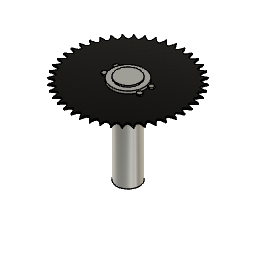
Gear (Autodesk Fusion 360 design; units mm, degrees)
Autodesk Fusion 360 part; units mm, degrees
(part 1 of 4)
sketch "Sketch1" plane through (0, 0, 0) normal (0, 0, 1) x (1, 0, 0)
  line L0 (12.5, 86.6025) -> (12.5, 76.4853)
  line L1 (0, 87.5) -> (0, 77.5)
  spline S0 degree 5 poles (0, 87.5) (0.2426, 86.8577) (0.7286, 85.6271) (1.4594, 83.9437) (2.4376, 82.0293) (3.6674, 80.2243) (4.9048, 79.0612) (6.1503, 78.5945) (7.4045, 78.8575) (8.667, 79.8263) (9.9372, 81.4497) (10.959, 83.23) (11.7283, 84.8192) (12.2426, 85.9896) (12.5, 86.6025) knots 0 0 0 0 0 0 0.1 0.2 0.3 0.4 0.5 0.6 0.7 0.8 0.9 1 1 1 1 1 1
  arc A0 (12.5, 76.4853) -> (0, 77.5) centre (0, 0) ccw
  line L2 (12.5, 89) -> (12.5, 81) construction
  line L3 (6.25, 87.5341) -> (6.25, 78.7707) construction
  arc A1 (1.4878, 77.4857) -> (-11.0294, 76.7112) centre (0, 0) ccw
  line L4 (-12.4525, 86.6094) -> (-11.0294, 76.7112)
  spline S1 degree 5 poles (-12.4525, 86.6094) (-12.121, 86.0081) (-11.4649, 84.8592) (-10.5019, 83.2969) (-9.2612, 81.5413) (-7.787, 79.9297) (-6.3967, 78.9545) (-5.0974, 78.6698) (-3.8935, 79.1086) (-2.7817, 80.2473) (-1.7555, 82.0348) (-0.9974, 83.9425) (-0.4621, 85.6249) (-0.1196, 86.8566) (0.0479, 87.5) knots 0 0 0 0 0 0 0.1 0.2 0.3 0.4 0.5 0.6 0.7 0.8 0.9 1 1 1 1 1 1
  line L5 (0.0479, 87.5) -> (1.4878, 77.4857)
  arc A2 (-9.5547, 76.9088) -> (-21.8343, 74.3607) centre (0, 0) ccw
  line L6 (-24.6516, 83.9556) -> (-21.8343, 74.3607)
  spline S2 degree 5 poles (-24.6516, 83.9556) (-24.2378, 83.4077) (-23.4249, 82.3639) (-22.2494, 80.9545) (-20.7714, 79.3933) (-19.0829, 78.0079) (-17.568, 77.2405) (-16.2414, 77.1436) (-15.1122, 77.7493) (-14.1738, 79.0346) (-13.4124, 80.95) (-12.9335, 82.9461) (-12.6431, 84.6876) (-12.4794, 85.9555) (-12.4051, 86.6162) knots 0 0 0 0 0 0 0.1 0.2 0.3 0.4 0.5 0.6 0.7 0.8 0.9 1 1 1 1 1 1
  line L7 (-12.4051, 86.6162) -> (-9.5547, 76.9088)
  arc A3 (-20.4027, 74.7662) -> (-32.1947, 70.4965) centre (0, 0) ccw
  line L8 (-36.3488, 79.5928) -> (-32.1947, 70.4965)
  spline S3 degree 5 poles (-36.3488, 79.5928) (-35.8613, 79.1093) (-34.9081, 78.1918) (-33.544, 76.9641) (-31.8588, 75.6291) (-29.9904, 74.4981) (-28.3817, 73.9542) (-27.0548, 74.047) (-26.0232, 74.8073) (-25.2773, 76.213) (-24.7963, 78.2173) (-24.6064, 80.2612) (-24.5667, 82.0264) (-24.5851, 83.3046) (-24.6056, 83.9691) knots 0 0 0 0 0 0 0.1 0.2 0.3 0.4 0.5 0.6 0.7 0.8 0.9 1 1 1 1 1 1
  line L9 (-24.6056, 83.9691) -> (-20.4027, 74.7662)
  arc A4 (-30.8354, 71.1015) -> (-41.8997, 65.1971) centre (0, 0) ccw
  line L10 (-47.3061, 73.6097) -> (-41.8997, 65.1971)
  spline S4 degree 5 poles (-47.3061, 73.6097) (-46.7547, 73.2005) (-45.6806, 72.428) (-44.1557, 71.4069) (-42.2977, 70.3253) (-40.2873, 69.4718) (-38.6176, 69.1623) (-37.3174, 69.443) (-36.4045, 70.3423) (-35.8663, 71.8399) (-35.6754, 73.8923) (-35.7783, 75.9424) (-35.9902, 77.6952) (-36.1904, 78.9579) (-36.3052, 79.6127) knots 0 0 0 0 0 0 0.1 0.2 0.3 0.4 0.5 0.6 0.7 0.8 0.9 1 1 1 1 1 1
  line L11 (-36.3052, 79.6127) -> (-30.8354, 71.1015)
  arc A5 (-40.6403, 65.9895) -> (-50.7517, 58.5706) centre (0, 0) ccw
  line L12 (-57.3003, 66.1281) -> (-50.7517, 58.5706)
  spline S5 degree 5 poles (-57.3003, 66.1281) (-56.6963, 65.8015) (-55.5232, 65.1898) (-53.8685, 64.3961) (-51.8755, 63.5899) (-49.7641, 63.0312) (-48.0673, 62.9624) (-46.8203, 63.4254) (-46.0448, 64.4455) (-45.7251, 66.0044) (-45.8282, 68.063) (-46.2218, 70.0777) (-46.681, 71.7825) (-47.0589, 73.0038) (-47.2657, 73.6356) knots 0 0 0 0 0 0 0.1 0.2 0.3 0.4 0.5 0.6 0.7 0.8 0.9 1 1 1 1 1 1
  line L13 (-47.2657, 73.6356) -> (-40.6403, 65.9895)
  arc A6 (-49.618, 59.5341) -> (-58.5706, 50.7517) centre (0, 0) ccw
  line L14 (-66.1281, 57.3003) -> (-58.5706, 50.7517)
  spline S6 degree 5 poles (-66.1281, 57.3003) (-65.4837, 57.063) (-64.2355, 56.6244) (-62.4847, 56.0743) (-60.3973, 55.56) (-58.2279, 55.3074) (-56.5386, 55.4809) (-55.3701, 56.1166) (-54.7476, 57.2366) (-54.6531, 58.8252) (-55.0481, 60.8482) (-55.7245, 62.7863) (-56.4216, 64.4084) (-56.9694, 65.5635) (-57.2641, 66.1595) knots 0 0 0 0 0 0 0.1 0.2 0.3 0.4 0.5 0.6 0.7 0.8 0.9 1 1 1 1 1 1
  line L15 (-57.2641, 66.1595) -> (-49.618, 59.5341)
  arc A7 (-57.5855, 51.8667) -> (-65.1971, 41.8997) centre (0, 0) ccw
  line L16 (-73.6097, 47.3061) -> (-65.1971, 41.8997)
  spline S7 degree 5 poles (-73.6097, 47.3061) (-72.9381, 47.1629) (-71.6402, 46.9064) (-69.8289, 46.6111) (-67.6896, 46.3991) (-65.5062, 46.4578) (-63.8588, 46.8699) (-62.7928, 47.6654) (-62.336, 48.8627) (-62.4685, 50.4485) (-63.1474, 52.3947) (-64.0927, 54.2168) (-65.0136, 55.7232) (-65.7202, 56.7886) (-66.0967, 57.3365) knots 0 0 0 0 0 0 0.1 0.2 0.3 0.4 0.5 0.6 0.7 0.8 0.9 1 1 1 1 1 1
  line L17 (-66.0967, 57.3365) -> (-57.5855, 51.8667)
  arc A8 (-64.3808, 43.1435) -> (-70.4965, 32.1947) centre (0, 0) ccw
  line L18 (-79.5928, 36.3488) -> (-70.4965, 32.1947)
  spline S8 degree 5 poles (-79.5928, 36.3488) (-78.9077, 36.3027) (-77.5865, 36.2335) (-75.7516, 36.1989) (-73.6038, 36.2936) (-71.4511, 36.6624) (-69.8791, 37.3048) (-68.9371, 38.2439) (-68.6554, 39.494) (-69.0122, 41.0448) (-69.9612, 42.8746) (-71.1562, 44.5436) (-72.2821, 45.9036) (-73.1331, 46.8576) (-73.5838, 47.3464) knots 0 0 0 0 0 0 0.1 0.2 0.3 0.4 0.5 0.6 0.7 0.8 0.9 1 1 1 1 1 1
  line L19 (-73.5838, 47.3464) -> (-64.3808, 43.1435)
  arc A9 (-69.8654, 33.5421) -> (-74.3607, 21.8343) centre (0, 0) ccw
  line L20 (-83.9556, 24.6516) -> (-74.3607, 21.8343)
  spline S9 degree 5 poles (-83.9556, 24.6516) (-83.271, 24.7034) (-81.9534, 24.823) (-80.1322, 25.0499) (-78.0198, 25.4492) (-75.9415, 26.1207) (-74.4769, 26.9802) (-73.6781, 28.0438) (-73.5772, 29.3213) (-74.151, 30.8056) (-75.3508, 32.4817) (-76.7711, 33.9637) (-78.0791, 35.1496) (-79.0573, 35.9727) (-79.5729, 36.3924) knots 0 0 0 0 0 0 0.1 0.2 0.3 0.4 0.5 0.6 0.7 0.8 0.9 1 1 1 1 1 1
  line L21 (-79.5729, 36.3924) -> (-69.8654, 33.5421)
  arc A10 (-73.9278, 23.2578) -> (-76.7112, 11.0294) centre (0, 0) ccw
  line L22 (-86.6094, 12.4525) -> (-76.7112, 11.0294)
  spline S10 degree 5 poles (-86.6094, 12.4525) (-85.939, 12.6013) (-84.6519, 12.9072) (-82.8816, 13.3909) (-80.8475, 14.0868) (-78.8858, 15.0472) (-77.5585, 16.1064) (-76.9192, 17.2729) (-77.0011, 18.5517) (-77.7804, 19.9392) (-79.2064, 21.4275) (-80.8232, 22.6923) (-82.2867, 23.68) (-83.372, 24.3555) (-83.9421, 24.6976) knots 0 0 0 0 0 0 0.1 0.2 0.3 0.4 0.5 0.6 0.7 0.8 0.9 1 1 1 1 1 1
  line L23 (-83.9421, 24.6976) -> (-73.9278, 23.2578)
  arc A11 (-76.4853, 12.5) -> (-77.5, 0) centre (0, 0) ccw
  line L24 (-87.5, 0) -> (-77.5, 0)
  spline S11 degree 5 poles (-87.5, 0) (-86.8577, 0.2426) (-85.6271, 0.7286) (-83.9437, 1.4594) (-82.0293, 2.4376) (-80.2243, 3.6674) (-79.0612, 4.9048) (-78.5945, 6.1503) (-78.8575, 7.4045) (-79.8263, 8.667) (-81.4497, 9.9372) (-83.23, 10.959) (-84.8192, 11.7283) (-85.9896, 12.2426) (-86.6025, 12.5) knots 0 0 0 0 0 0 0.1 0.2 0.3 0.4 0.5 0.6 0.7 0.8 0.9 1 1 1 1 1 1
  line L25 (-86.6025, 12.5) -> (-76.4853, 12.5)
  arc A12 (-77.4857, 1.4878) -> (-76.7112, -11.0294) centre (0, 0) ccw
  line L26 (-86.6094, -12.4525) -> (-76.7112, -11.0294)
  spline S12 degree 5 poles (-86.6094, -12.4525) (-86.0081, -12.121) (-84.8592, -11.4649) (-83.2969, -10.5019) (-81.5413, -9.2612) (-79.9297, -7.787) (-78.9545, -6.3967) (-78.6698, -5.0974) (-79.1086, -3.8935) (-80.2473, -2.7817) (-82.0348, -1.7555) (-83.9425, -0.9974) (-85.6249, -0.4621) (-86.8566, -0.1196) (-87.5, 0.0479) knots 0 0 0 0 0 0 0.1 0.2 0.3 0.4 0.5 0.6 0.7 0.8 0.9 1 1 1 1 1 1
  line L27 (-87.5, 0.0479) -> (-77.4857, 1.4878)
  arc A13 (-76.9088, -9.5547) -> (-74.3607, -21.8343) centre (0, 0) ccw
  line L28 (-83.9556, -24.6516) -> (-74.3607, -21.8343)
  spline S13 degree 5 poles (-83.9556, -24.6516) (-83.4077, -24.2378) (-82.3639, -23.4249) (-80.9545, -22.2494) (-79.3933, -20.7714) (-78.0079, -19.0829) (-77.2405, -17.568) (-77.1436, -16.2414) (-77.7493, -15.1122) (-79.0346, -14.1738) (-80.95, -13.4124) (-82.9461, -12.9335) (-84.6876, -12.6431) (-85.9555, -12.4794) (-86.6162, -12.4051) knots 0 0 0 0 0 0 0.1 0.2 0.3 0.4 0.5 0.6 0.7 0.8 0.9 1 1 1 1 1 1
  line L29 (-86.6162, -12.4051) -> (-76.9088, -9.5547)
  arc A14 (-74.7662, -20.4027) -> (-70.4965, -32.1947) centre (0, 0) ccw
  line L30 (-79.5928, -36.3488) -> (-70.4965, -32.1947)
  spline S14 degree 5 poles (-79.5928, -36.3488) (-79.1093, -35.8613) (-78.1918, -34.9081) (-76.9641, -33.544) (-75.6291, -31.8588) (-74.4981, -29.9904) (-73.9542, -28.3817) (-74.047, -27.0548) (-74.8073, -26.0232) (-76.213, -25.2773) (-78.2173, -24.7963) (-80.2612, -24.6064) (-82.0264, -24.5667) (-83.3046, -24.5851) (-83.9691, -24.6056) knots 0 0 0 0 0 0 0.1 0.2 0.3 0.4 0.5 0.6 0.7 0.8 0.9 1 1 1 1 1 1
  line L31 (-83.9691, -24.6056) -> (-74.7662, -20.4027)
  arc A15 (-71.1015, -30.8354) -> (-65.1971, -41.8997) centre (0, 0) ccw
  line L32 (-73.6097, -47.3061) -> (-65.1971, -41.8997)
  spline S15 degree 5 poles (-73.6097, -47.3061) (-73.2005, -46.7547) (-72.428, -45.6806) (-71.4069, -44.1557) (-70.3253, -42.2977) (-69.4718, -40.2873) (-69.1623, -38.6176) (-69.443, -37.3174) (-70.3423, -36.4045) (-71.8399, -35.8663) (-73.8923, -35.6754) (-75.9424, -35.7783) (-77.6952, -35.9902) (-78.9579, -36.1904) (-79.6127, -36.3052) knots 0 0 0 0 0 0 0.1 0.2 0.3 0.4 0.5 0.6 0.7 0.8 0.9 1 1 1 1 1 1
  line L33 (-79.6127, -36.3052) -> (-71.1015, -30.8354)
  arc A16 (-65.9895, -40.6403) -> (-58.5706, -50.7517) centre (0, 0) ccw
  line L34 (-66.1281, -57.3003) -> (-58.5706, -50.7517)
  spline S16 degree 5 poles (-66.1281, -57.3003) (-65.8015, -56.6963) (-65.1898, -55.5232) (-64.3961, -53.8685) (-63.5899, -51.8755) (-63.0312, -49.7641) (-62.9624, -48.0673) (-63.4254, -46.8203) (-64.4455, -46.0448) (-66.0044, -45.7251) (-68.063, -45.8282) (-70.0777, -46.2218) (-71.7825, -46.681) (-73.0038, -47.0589) (-73.6356, -47.2657) knots 0 0 0 0 0 0 0.1 0.2 0.3 0.4 0.5 0.6 0.7 0.8 0.9 1 1 1 1 1 1
  line L35 (-73.6356, -47.2657) -> (-65.9895, -40.6403)
  arc A17 (-59.5341, -49.618) -> (-50.7517, -58.5706) centre (0, 0) ccw
  line L36 (-57.3003, -66.1281) -> (-50.7517, -58.5706)
  spline S17 degree 5 poles (-57.3003, -66.1281) (-57.063, -65.4837) (-56.6244, -64.2355) (-56.0743, -62.4847) (-55.56, -60.3973) (-55.3074, -58.2279) (-55.4809, -56.5386) (-56.1166, -55.3701) (-57.2366, -54.7476) (-58.8252, -54.6531) (-60.8482, -55.0481) (-62.7863, -55.7245) (-64.4084, -56.4216) (-65.5635, -56.9694) (-66.1595, -57.2641) knots 0 0 0 0 0 0 0.1 0.2 0.3 0.4 0.5 0.6 0.7 0.8 0.9 1 1 1 1 1 1
  line L37 (-66.1595, -57.2641) -> (-59.5341, -49.618)
  arc A18 (-51.8667, -57.5855) -> (-41.8997, -65.1971) centre (0, 0) ccw
  line L38 (-47.3061, -73.6097) -> (-41.8997, -65.1971)
  spline S18 degree 5 poles (-47.3061, -73.6097) (-47.1629, -72.9381) (-46.9064, -71.6402) (-46.6111, -69.8289) (-46.3991, -67.6896) (-46.4578, -65.5062) (-46.8699, -63.8588) (-47.6654, -62.7928) (-48.8627, -62.336) (-50.4485, -62.4685) (-52.3947, -63.1474) (-54.2168, -64.0927) (-55.7232, -65.0136) (-56.7886, -65.7202) (-57.3365, -66.0967) knots 0 0 0 0 0 0 0.1 0.2 0.3 0.4 0.5 0.6 0.7 0.8 0.9 1 1 1 1 1 1
  line L39 (-57.3365, -66.0967) -> (-51.8667, -57.5855)
  arc A19 (-43.1435, -64.3808) -> (-32.1947, -70.4965) centre (0, 0) ccw
  line L40 (-36.3488, -79.5928) -> (-32.1947, -70.4965)
  spline S19 degree 5 poles (-36.3488, -79.5928) (-36.3027, -78.9077) (-36.2335, -77.5865) (-36.1989, -75.7516) (-36.2936, -73.6038) (-36.6624, -71.4511) (-37.3048, -69.8791) (-38.2439, -68.9371) (-39.494, -68.6554) (-41.0448, -69.0122) (-42.8746, -69.9612) (-44.5436, -71.1562) (-45.9036, -72.2821) (-46.8576, -73.1331) (-47.3464, -73.5838) knots 0 0 0 0 0 0 0.1 0.2 0.3 0.4 0.5 0.6 0.7 0.8 0.9 1 1 1 1 1 1
  line L41 (-47.3464, -73.5838) -> (-43.1435, -64.3808)
  arc A20 (-33.5421, -69.8654) -> (-21.8343, -74.3607) centre (0, 0) ccw
  line L42 (-24.6516, -83.9556) -> (-21.8343, -74.3607)
  spline S20 degree 5 poles (-24.6516, -83.9556) (-24.7034, -83.271) (-24.823, -81.9534) (-25.0499, -80.1322) (-25.4492, -78.0198) (-26.1207, -75.9415) (-26.9802, -74.4769) (-28.0438, -73.6781) (-29.3213, -73.5772) (-30.8056, -74.151) (-32.4817, -75.3508) (-33.9637, -76.7711) (-35.1496, -78.0791) (-35.9727, -79.0573) (-36.3924, -79.5729) knots 0 0 0 0 0 0 0.1 0.2 0.3 0.4 0.5 0.6 0.7 0.8 0.9 1 1 1 1 1 1
  line L43 (-36.3924, -79.5729) -> (-33.5421, -69.8654)
  arc A21 (-23.2578, -73.9278) -> (-11.0294, -76.7112) centre (0, 0) ccw
  line L44 (-12.4525, -86.6094) -> (-11.0294, -76.7112)
  spline S21 degree 5 poles (-12.4525, -86.6094) (-12.6013, -85.939) (-12.9072, -84.6519) (-13.3909, -82.8816) (-14.0868, -80.8475) (-15.0472, -78.8858) (-16.1064, -77.5585) (-17.2729, -76.9192) (-18.5517, -77.0011) (-19.9392, -77.7804) (-21.4275, -79.2064) (-22.6923, -80.8232) (-23.68, -82.2867) (-24.3555, -83.372) (-24.6976, -83.9421) knots 0 0 0 0 0 0 0.1 0.2 0.3 0.4 0.5 0.6 0.7 0.8 0.9 1 1 1 1 1 1
  line L45 (-24.6976, -83.9421) -> (-23.2578, -73.9278)
  arc A22 (-12.5, -76.4853) -> (0, -77.5) centre (0, 0) ccw
  line L46 (0, -87.5) -> (0, -77.5)
  spline S22 degree 5 poles (0, -87.5) (-0.2426, -86.8577) (-0.7286, -85.6271) (-1.4594, -83.9437) (-2.4376, -82.0293) (-3.6674, -80.2243) (-4.9048, -79.0612) (-6.1503, -78.5945) (-7.4045, -78.8575) (-8.667, -79.8263) (-9.9372, -81.4497) (-10.959, -83.23) (-11.7283, -84.8192) (-12.2426, -85.9896) (-12.5, -86.6025) knots 0 0 0 0 0 0 0.1 0.2 0.3 0.4 0.5 0.6 0.7 0.8 0.9 1 1 1 1 1 1
  line L47 (-12.5, -86.6025) -> (-12.5, -76.4853)
  arc A23 (-1.4878, -77.4857) -> (11.0294, -76.7112) centre (0, 0) ccw
  line L48 (12.4525, -86.6094) -> (11.0294, -76.7112)
  spline S23 degree 5 poles (12.4525, -86.6094) (12.121, -86.0081) (11.4649, -84.8592) (10.5019, -83.2969) (9.2612, -81.5413) (7.787, -79.9297) (6.3967, -78.9545) (5.0974, -78.6698) (3.8935, -79.1086) (2.7817, -80.2473) (1.7555, -82.0348) (0.9974, -83.9425) (0.4621, -85.6249) (0.1196, -86.8566) (-0.0479, -87.5) knots 0 0 0 0 0 0 0.1 0.2 0.3 0.4 0.5 0.6 0.7 0.8 0.9 1 1 1 1 1 1
  line L49 (-0.0479, -87.5) -> (-1.4878, -77.4857)
  arc A24 (9.5547, -76.9088) -> (21.8343, -74.3607) centre (0, 0) ccw
  line L50 (24.6516, -83.9556) -> (21.8343, -74.3607)
  spline S24 degree 5 poles (24.6516, -83.9556) (24.2378, -83.4077) (23.4249, -82.3639) (22.2494, -80.9545) (20.7714, -79.3933) (19.0829, -78.0079) (17.568, -77.2405) (16.2414, -77.1436) (15.1122, -77.7493) (14.1738, -79.0346) (13.4124, -80.95) (12.9335, -82.9461) (12.6431, -84.6876) (12.4794, -85.9555) (12.4051, -86.6162) knots 0 0 0 0 0 0 0.1 0.2 0.3 0.4 0.5 0.6 0.7 0.8 0.9 1 1 1 1 1 1
  line L51 (12.4051, -86.6162) -> (9.5547, -76.9088)
  arc A25 (20.4027, -74.7662) -> (32.1947, -70.4965) centre (0, 0) ccw
  line L52 (36.3488, -79.5928) -> (32.1947, -70.4965)
  spline S25 degree 5 poles (36.3488, -79.5928) (35.8613, -79.1093) (34.9081, -78.1918) (33.544, -76.9641) (31.8588, -75.6291) (29.9904, -74.4981) (28.3817, -73.9542) (27.0548, -74.047) (26.0232, -74.8073) (25.2773, -76.213) (24.7963, -78.2173) (24.6064, -80.2612) (24.5667, -82.0264) (24.5851, -83.3046) (24.6056, -83.9691) knots 0 0 0 0 0 0 0.1 0.2 0.3 0.4 0.5 0.6 0.7 0.8 0.9 1 1 1 1 1 1
  line L53 (24.6056, -83.9691) -> (20.4027, -74.7662)
  arc A26 (30.8354, -71.1015) -> (41.8997, -65.1971) centre (0, 0) ccw
  line L54 (47.3061, -73.6097) -> (41.8997, -65.1971)
  spline S26 degree 5 poles (47.3061, -73.6097) (46.7547, -73.2005) (45.6806, -72.428) (44.1557, -71.4069) (42.2977, -70.3253) (40.2873, -69.4718) (38.6176, -69.1623) (37.3174, -69.443) (36.4045, -70.3423) (35.8663, -71.8399) (35.6754, -73.8923) (35.7783, -75.9424) (35.9902, -77.6952) (36.1904, -78.9579) (36.3052, -79.6127) knots 0 0 0 0 0 0 0.1 0.2 0.3 0.4 0.5 0.6 0.7 0.8 0.9 1 1 1 1 1 1
  line L55 (36.3052, -79.6127) -> (30.8354, -71.1015)
  arc A27 (40.6403, -65.9895) -> (50.7517, -58.5706) centre (0, 0) ccw
  line L56 (57.3003, -66.1281) -> (50.7517, -58.5706)
  spline S27 degree 5 poles (57.3003, -66.1281) (56.6963, -65.8015) (55.5232, -65.1898) (53.8685, -64.3961) (51.8755, -63.5899) (49.7641, -63.0312) (48.0673, -62.9624) (46.8203, -63.4254) (46.0448, -64.4455) (45.7251, -66.0044) (45.8282, -68.063) (46.2218, -70.0777) (46.681, -71.7825) (47.0589, -73.0038) (47.2657, -73.6356) knots 0 0 0 0 0 0 0.1 0.2 0.3 0.4 0.5 0.6 0.7 0.8 0.9 1 1 1 1 1 1
  line L57 (47.2657, -73.6356) -> (40.6403, -65.9895)
  arc A28 (49.618, -59.5341) -> (58.5706, -50.7517) centre (0, 0) ccw
  line L58 (66.1281, -57.3003) -> (58.5706, -50.7517)
  spline S28 degree 5 poles (66.1281, -57.3003) (65.4837, -57.063) (64.2355, -56.6244) (62.4847, -56.0743) (60.3973, -55.56) (58.2279, -55.3074) (56.5386, -55.4809) (55.3701, -56.1166) (54.7476, -57.2366) (54.6531, -58.8252) (55.0481, -60.8482) (55.7245, -62.7863) (56.4216, -64.4084) (56.9694, -65.5635) (57.2641, -66.1595) knots 0 0 0 0 0 0 0.1 0.2 0.3 0.4 0.5 0.6 0.7 0.8 0.9 1 1 1 1 1 1
  line L59 (57.2641, -66.1595) -> (49.618, -59.5341)
  arc A29 (57.5855, -51.8667) -> (65.1971, -41.8997) centre (0, 0) ccw
  line L60 (73.6097, -47.3061) -> (65.1971, -41.8997)
  spline S29 degree 5 poles (73.6097, -47.3061) (72.9381, -47.1629) (71.6402, -46.9064) (69.8289, -46.6111) (67.6896, -46.3991) (65.5062, -46.4578) (63.8588, -46.8699) (62.7928, -47.6654) (62.336, -48.8627) (62.4685, -50.4485) (63.1474, -52.3947) (64.0927, -54.2168) (65.0136, -55.7232) (65.7202, -56.7886) (66.0967, -57.3365) knots 0 0 0 0 0 0 0.1 0.2 0.3 0.4 0.5 0.6 0.7 0.8 0.9 1 1 1 1 1 1
  line L61 (66.0967, -57.3365) -> (57.5855, -51.8667)
  arc A30 (64.3808, -43.1435) -> (70.4965, -32.1947) centre (0, 0) ccw
  line L62 (79.5928, -36.3488) -> (70.4965, -32.1947)
  spline S30 degree 5 poles (79.5928, -36.3488) (78.9077, -36.3027) (77.5865, -36.2335) (75.7516, -36.1989) (73.6038, -36.2936) (71.4511, -36.6624) (69.8791, -37.3048) (68.9371, -38.2439) (68.6554, -39.494) (69.0122, -41.0448) (69.9612, -42.8746) (71.1562, -44.5436) (72.2821, -45.9036) (73.1331, -46.8576) (73.5838, -47.3464) knots 0 0 0 0 0 0 0.1 0.2 0.3 0.4 0.5 0.6 0.7 0.8 0.9 1 1 1 1 1 1
  line L63 (73.5838, -47.3464) -> (64.3808, -43.1435)
  arc A31 (69.8654, -33.5421) -> (74.3607, -21.8343) centre (0, 0) ccw
  line L64 (83.9556, -24.6516) -> (74.3607, -21.8343)
  spline S31 degree 5 poles (83.9556, -24.6516) (83.271, -24.7034) (81.9534, -24.823) (80.1322, -25.0499) (78.0198, -25.4492) (75.9415, -26.1207) (74.4769, -26.9802) (73.6781, -28.0438) (73.5772, -29.3213) (74.151, -30.8056) (75.3508, -32.4817) (76.7711, -33.9637) (78.0791, -35.1496) (79.0573, -35.9727) (79.5729, -36.3924) knots 0 0 0 0 0 0 0.1 0.2 0.3 0.4 0.5 0.6 0.7 0.8 0.9 1 1 1 1 1 1
  line L65 (79.5729, -36.3924) -> (69.8654, -33.5421)
  arc A32 (73.9278, -23.2578) -> (76.7112, -11.0294) centre (0, 0) ccw
  line L66 (86.6094, -12.4525) -> (76.7112, -11.0294)
  spline S32 degree 5 poles (86.6094, -12.4525) (85.939, -12.6013) (84.6519, -12.9072) (82.8816, -13.3909) (80.8475, -14.0868) (78.8858, -15.0472) (77.5585, -16.1064) (76.9192, -17.2729) (77.0011, -18.5517) (77.7804, -19.9392) (79.2064, -21.4275) (80.8232, -22.6923) (82.2867, -23.68) (83.372, -24.3555) (83.9421, -24.6976) knots 0 0 0 0 0 0 0.1 0.2 0.3 0.4 0.5 0.6 0.7 0.8 0.9 1 1 1 1 1 1
  line L67 (83.9421, -24.6976) -> (73.9278, -23.2578)
  arc A33 (76.4853, -12.5) -> (77.5, 0) centre (0, 0) ccw
  line L68 (87.5, 0) -> (77.5, 0)
  spline S33 degree 5 poles (87.5, 0) (86.8577, -0.2426) (85.6271, -0.7286) (83.9437, -1.4594) (82.0293, -2.4376) (80.2243, -3.6674) (79.0612, -4.9048) (78.5945, -6.1503) (78.8575, -7.4045) (79.8263, -8.667) (81.4497, -9.9372) (83.23, -10.959) (84.8192, -11.7283) (85.9896, -12.2426) (86.6025, -12.5) knots 0 0 0 0 0 0 0.1 0.2 0.3 0.4 0.5 0.6 0.7 0.8 0.9 1 1 1 1 1 1
  line L69 (86.6025, -12.5) -> (76.4853, -12.5)
  arc A34 (77.4857, -1.4878) -> (76.7112, 11.0294) centre (0, 0) ccw
  line L70 (86.6094, 12.4525) -> (76.7112, 11.0294)
  spline S34 degree 5 poles (86.6094, 12.4525) (86.0081, 12.121) (84.8592, 11.4649) (83.2969, 10.5019) (81.5413, 9.2612) (79.9297, 7.787) (78.9545, 6.3967) (78.6698, 5.0974) (79.1086, 3.8935) (80.2473, 2.7817) (82.0348, 1.7555) (83.9425, 0.9974) (85.6249, 0.4621) (86.8566, 0.1196) (87.5, -0.0479) knots 0 0 0 0 0 0 0.1 0.2 0.3 0.4 0.5 0.6 0.7 0.8 0.9 1 1 1 1 1 1
  line L71 (87.5, -0.0479) -> (77.4857, -1.4878)
  arc A35 (76.9088, 9.5547) -> (74.3607, 21.8343) centre (0, 0) ccw
  line L72 (83.9556, 24.6516) -> (74.3607, 21.8343)
  spline S35 degree 5 poles (83.9556, 24.6516) (83.4077, 24.2378) (82.3639, 23.4249) (80.9545, 22.2494) (79.3933, 20.7714) (78.0079, 19.0829) (77.2405, 17.568) (77.1436, 16.2414) (77.7493, 15.1122) (79.0346, 14.1738) (80.95, 13.4124) (82.9461, 12.9335) (84.6876, 12.6431) (85.9555, 12.4794) (86.6162, 12.4051) knots 0 0 0 0 0 0 0.1 0.2 0.3 0.4 0.5 0.6 0.7 0.8 0.9 1 1 1 1 1 1
  line L73 (86.6162, 12.4051) -> (76.9088, 9.5547)
  arc A36 (74.7662, 20.4027) -> (70.4965, 32.1947) centre (0, 0) ccw
  line L74 (79.5928, 36.3488) -> (70.4965, 32.1947)
  spline S36 degree 5 poles (79.5928, 36.3488) (79.1093, 35.8613) (78.1918, 34.9081) (76.9641, 33.544) (75.6291, 31.8588) (74.4981, 29.9904) (73.9542, 28.3817) (74.047, 27.0548) (74.8073, 26.0232) (76.213, 25.2773) (78.2173, 24.7963) (80.2612, 24.6064) (82.0264, 24.5667) (83.3046, 24.5851) (83.9691, 24.6056) knots 0 0 0 0 0 0 0.1 0.2 0.3 0.4 0.5 0.6 0.7 0.8 0.9 1 1 1 1 1 1
  line L75 (83.9691, 24.6056) -> (74.7662, 20.4027)
  arc A37 (71.1015, 30.8354) -> (65.1971, 41.8997) centre (0, 0) ccw
  line L76 (73.6097, 47.3061) -> (65.1971, 41.8997)
  spline S37 degree 5 poles (73.6097, 47.3061) (73.2005, 46.7547) (72.428, 45.6806) (71.4069, 44.1557) (70.3253, 42.2977) (69.4718, 40.2873) (69.1623, 38.6176) (69.443, 37.3174) (70.3423, 36.4045) (71.8399, 35.8663) (73.8923, 35.6754) (75.9424, 35.7783) (77.6952, 35.9902) (78.9579, 36.1904) (79.6127, 36.3052) knots 0 0 0 0 0 0 0.1 0.2 0.3 0.4 0.5 0.6 0.7 0.8 0.9 1 1 1 1 1 1
  line L77 (79.6127, 36.3052) -> (71.1015, 30.8354)
  arc A38 (65.9895, 40.6403) -> (58.5706, 50.7517) centre (0, 0) ccw
  line L78 (66.1281, 57.3003) -> (58.5706, 50.7517)
  spline S38 degree 5 poles (66.1281, 57.3003) (65.8015, 56.6963) (65.1898, 55.5232) (64.3961, 53.8685) (63.5899, 51.8755) (63.0312, 49.7641) (62.9624, 48.0673) (63.4254, 46.8203) (64.4455, 46.0448) (66.0044, 45.7251) (68.063, 45.8282) (70.0777, 46.2218) (71.7825, 46.681) (73.0038, 47.0589) (73.6356, 47.2657) knots 0 0 0 0 0 0 0.1 0.2 0.3 0.4 0.5 0.6 0.7 0.8 0.9 1 1 1 1 1 1
  line L79 (73.6356, 47.2657) -> (65.9895, 40.6403)
  arc A39 (59.5341, 49.618) -> (50.7517, 58.5706) centre (0, 0) ccw
  line L80 (57.3003, 66.1281) -> (50.7517, 58.5706)
  spline S39 degree 5 poles (57.3003, 66.1281) (57.063, 65.4837) (56.6244, 64.2355) (56.0743, 62.4847) (55.56, 60.3973) (55.3074, 58.2279) (55.4809, 56.5386) (56.1166, 55.3701) (57.2366, 54.7476) (58.8252, 54.6531) (60.8482, 55.0481) (62.7863, 55.7245) (64.4084, 56.4216) (65.5635, 56.9694) (66.1595, 57.2641) knots 0 0 0 0 0 0 0.1 0.2 0.3 0.4 0.5 0.6 0.7 0.8 0.9 1 1 1 1 1 1
  line L81 (66.1595, 57.2641) -> (59.5341, 49.618)
  arc A40 (51.8667, 57.5855) -> (41.8997, 65.1971) centre (0, 0) ccw
  line L82 (47.3061, 73.6097) -> (41.8997, 65.1971)
  spline S40 degree 5 poles (47.3061, 73.6097) (47.1629, 72.9381) (46.9064, 71.6402) (46.6111, 69.8289) (46.3991, 67.6896) (46.4578, 65.5062) (46.8699, 63.8588) (47.6654, 62.7928) (48.8627, 62.336) (50.4485, 62.4685) (52.3947, 63.1474) (54.2168, 64.0927) (55.7232, 65.0136) (56.7886, 65.7202) (57.3365, 66.0967) knots 0 0 0 0 0 0 0.1 0.2 0.3 0.4 0.5 0.6 0.7 0.8 0.9 1 1 1 1 1 1
  line L83 (57.3365, 66.0967) -> (51.8667, 57.5855)
  arc A41 (43.1435, 64.3808) -> (32.1947, 70.4965) centre (0, 0) ccw
  line L84 (36.3488, 79.5928) -> (32.1947, 70.4965)
  spline S41 degree 5 poles (36.3488, 79.5928) (36.3027, 78.9077) (36.2335, 77.5865) (36.1989, 75.7516) (36.2936, 73.6038) (36.6624, 71.4511) (37.3048, 69.8791) (38.2439, 68.9371) (39.494, 68.6554) (41.0448, 69.0122) (42.8746, 69.9612) (44.5436, 71.1562) (45.9036, 72.2821) (46.8576, 73.1331) (47.3464, 73.5838) knots 0 0 0 0 0 0 0.1 0.2 0.3 0.4 0.5 0.6 0.7 0.8 0.9 1 1 1 1 1 1
  line L85 (47.3464, 73.5838) -> (43.1435, 64.3808)
  arc A42 (33.5421, 69.8654) -> (21.8343, 74.3607) centre (0, 0) ccw
  line L86 (24.6516, 83.9556) -> (21.8343, 74.3607)
  spline S42 degree 5 poles (24.6516, 83.9556) (24.7034, 83.271) (24.823, 81.9534) (25.0499, 80.1322) (25.4492, 78.0198) (26.1207, 75.9415) (26.9802, 74.4769) (28.0438, 73.6781) (29.3213, 73.5772) (30.8056, 74.151) (32.4817, 75.3508) (33.9637, 76.7711) (35.1496, 78.0791) (35.9727, 79.0573) (36.3924, 79.5729) knots 0 0 0 0 0 0 0.1 0.2 0.3 0.4 0.5 0.6 0.7 0.8 0.9 1 1 1 1 1 1
  line L87 (36.3924, 79.5729) -> (33.5421, 69.8654)
  arc A43 (23.2578, 73.9278) -> (11.0294, 76.7112) centre (0, 0) ccw
  line L88 (12.4525, 86.6094) -> (11.0294, 76.7112)
  spline S43 degree 5 poles (12.4525, 86.6094) (12.6013, 85.939) (12.9072, 84.6519) (13.3909, 82.8816) (14.0868, 80.8475) (15.0472, 78.8858) (16.1064, 77.5585) (17.2729, 76.9192) (18.5517, 77.0011) (19.9392, 77.7804) (21.4275, 79.2064) (22.6923, 80.8232) (23.68, 82.2867) (24.3555, 83.372) (24.6976, 83.9421) knots 0 0 0 0 0 0 0.1 0.2 0.3 0.4 0.5 0.6 0.7 0.8 0.9 1 1 1 1 1 1
  line L89 (24.6976, 83.9421) -> (23.2578, 73.9278)
  point P0 (6.25, 78.7707)
  point P1 (-5.0239, 78.8584)
  point P2 (-16.1954, 77.3408)
  point P3 (-27.0373, 74.2487)
  point P4 (-37.3288, 69.6452)
  point P5 (-46.8604, 63.6238)
  point P6 (-55.4381, 56.3073)
  point P7 (-62.8872, 47.8445)
  point P8 (-69.056, 38.4077)
  point P9 (-73.8191, 28.1891)
  point P10 (-77.0795, 17.3966)
  point P11 (-78.7707, 6.25)
  point P12 (-78.8584, -5.0239)
  point P13 (-77.3408, -16.1954)
  point P14 (-74.2487, -27.0373)
  point P15 (-69.6452, -37.3288)
  point P16 (-63.6238, -46.8604)
  point P17 (-56.3073, -55.4381)
  point P18 (-47.8445, -62.8872)
  point P19 (-38.4077, -69.056)
  point P20 (-28.1891, -73.8191)
  point P21 (-17.3966, -77.0795)
  point P22 (-6.25, -78.7707)
  point P23 (5.0239, -78.8584)
  point P24 (16.1954, -77.3408)
  point P25 (27.0373, -74.2487)
  point P26 (37.3288, -69.6452)
  point P27 (46.8604, -63.6238)
  point P28 (55.4381, -56.3073)
  point P29 (62.8872, -47.8445)
  point P30 (69.056, -38.4077)
  point P31 (73.8191, -28.1891)
  point P32 (77.0795, -17.3966)
  point P33 (78.7707, -6.25)
  point P34 (78.8584, 5.0239)
  point P35 (77.3408, 16.1954)
  point P36 (74.2487, 27.0373)
  point P37 (69.6452, 37.3288)
  point P38 (63.6238, 46.8604)
  point P39 (56.3073, 55.4381)
  point P40 (47.8445, 62.8872)
  point P41 (38.4077, 69.056)
  point P42 (28.1891, 73.8191)
  point P43 (17.3966, 77.0795)
  dimension "d3" = 87.5
  dimension "d7" = 360
  constraint vertical L1
  constraint vertical L2
  constraint coincident L0.start L2
  constraint coincident L0.end L2
  constraint vertical L3
  constraint coincident P0 L3.end
  measures "d3" distance of L1.start A0.centre
extrude "Extrude1" add sketch "Sketch1" along normal blind 2 makes body 1
sketch "Sketch1 (2)" plane through (0, 0, 2) normal (0, 0, 1) x (-1, 0, 0) in component "Gear "
  line L0 (-24.6516, -83.9556) -> (-24.6001, -83.7803)
  spline S0 degree 5 poles (-24.6001, -83.7803) (-24.2785, -83.2487) (-23.6237, -82.2035) (-22.6562, -80.7772) (-21.4105, -79.1902) (-19.9392, -77.7804) (-18.5517, -77.0011) (-17.2729, -76.9192) (-16.1064, -77.5585) (-15.0472, -78.8858) (-14.099, -80.8225) (-13.4131, -82.817) (-12.938, -84.5397) (-12.6403, -85.776) (-12.5, -86.3974) knots -0.994293 -0.994293 -0.994293 -0.994293 -0.994293 -0.994293 -0.9 -0.8 -0.7 -0.6 -0.5 -0.4 -0.3 -0.2 -0.1 -0.006357 -0.006357 -0.006357 -0.006357 -0.006357 -0.006357
  line L1 (-12.5, -86.3974) -> (-12.5, -86.6025)
  line L2 (-12.5, -86.6025) -> (-12.47, -86.5312)
  line L3 (-12.47, -86.5312) -> (-12.4525, -86.6094)
  line L4 (-12.4525, -86.6094) -> (-12.4265, -86.4285)
  spline S1 degree 5 poles (-12.4265, -86.4285) (-12.1839, -85.8565) (-11.6844, -84.7287) (-10.9298, -83.1793) (-9.9227, -81.4312) (-8.667, -79.8263) (-7.4045, -78.8575) (-6.1503, -78.5945) (-4.9048, -79.0612) (-3.6674, -80.2243) (-2.4533, -82.0064) (-1.4905, -83.883) (-0.775, -85.5204) (-0.3044, -86.7019) (-0.0771, -87.2969) knots -0.994293 -0.994293 -0.994293 -0.994293 -0.994293 -0.994293 -0.9 -0.8 -0.7 -0.6 -0.5 -0.4 -0.3 -0.2 -0.1 -0.006357 -0.006357 -0.006357 -0.006357 -0.006357 -0.006357
  line L5 (-0.0771, -87.2969) -> (-0.0479, -87.5)
  line L6 (-0.0479, -87.5) -> (-0.0284, -87.4251)
  line L7 (-0.0284, -87.4251) -> (0, -87.5)
  line L8 (0, -87.5) -> (0, -87.3173)
  spline S2 degree 5 poles (0, -87.3173) (0.1588, -86.7166) (0.4926, -85.5292) (1.0191, -83.8882) (1.7672, -82.0144) (2.7817, -80.2473) (3.8935, -79.1086) (5.0974, -78.6698) (6.3967, -78.9545) (7.787, -79.9297) (9.2424, -81.5208) (10.4625, -83.2413) (11.4037, -84.7603) (12.0376, -85.8627) (12.3473, -86.4193) knots -0.994293 -0.994293 -0.994293 -0.994293 -0.994293 -0.994293 -0.9 -0.8 -0.7 -0.6 -0.5 -0.4 -0.3 -0.2 -0.1 -0.006357 -0.006357 -0.006357 -0.006357 -0.006357 -0.006357
  line L9 (12.3473, -86.4193) -> (12.4051, -86.6162)
  line L10 (12.4051, -86.6162) -> (12.4138, -86.5392)
  line L11 (12.4138, -86.5392) -> (12.4525, -86.6094)
  line L12 (12.4525, -86.6094) -> (12.4265, -86.4285)
  spline S3 degree 5 poles (12.4265, -86.4285) (12.4982, -85.8113) (12.6597, -84.5885) (12.9472, -82.8893) (13.4211, -80.9282) (14.1738, -79.0346) (15.1122, -77.7493) (16.2414, -77.1436) (17.568, -77.2405) (19.0829, -78.0079) (20.75, -79.3757) (22.2025, -80.905) (23.3503, -82.2746) (24.1346, -83.2756) (24.5204, -83.7825) knots -0.994293 -0.994293 -0.994293 -0.994293 -0.994293 -0.994293 -0.9 -0.8 -0.7 -0.6 -0.5 -0.4 -0.3 -0.2 -0.1 -0.006357 -0.006357 -0.006357 -0.006357 -0.006357 -0.006357
  line L13 (24.5204, -83.7825) -> (24.6056, -83.9691)
  line L14 (24.6056, -83.9691) -> (24.6033, -83.8917)
  line L15 (24.6033, -83.8917) -> (24.6516, -83.9556)
  line L16 (24.6516, -83.9556) -> (24.6001, -83.7803)
  spline S4 degree 5 poles (24.6001, -83.7803) (24.5832, -83.1592) (24.569, -81.9259) (24.6118, -80.203) (24.8018, -78.1944) (25.2773, -76.213) (26.0232, -74.8073) (27.0548, -74.047) (28.3817, -73.9542) (29.9904, -74.4981) (31.8351, -75.6147) (33.4905, -76.9218) (34.8215, -78.1141) (35.7403, -78.9933) (36.1943, -79.4401) knots -0.994293 -0.994293 -0.994293 -0.994293 -0.994293 -0.994293 -0.9 -0.8 -0.7 -0.6 -0.5 -0.4 -0.3 -0.2 -0.1 -0.006357 -0.006357 -0.006357 -0.006357 -0.006357 -0.006357
  line L17 (36.1943, -79.4401) -> (36.3052, -79.6127)
  line L18 (36.3052, -79.6127) -> (36.2919, -79.5364)
  line L19 (36.2919, -79.5364) -> (36.3488, -79.5928)
  line L20 (36.3488, -79.5928) -> (36.2729, -79.4266)
  spline S5 degree 5 poles (36.2729, -79.4266) (36.1678, -78.8142) (35.9782, -77.5954) (35.7754, -75.884) (35.6775, -73.8688) (35.8663, -71.8399) (36.4045, -70.3423) (37.3174, -69.443) (38.6176, -69.1623) (40.2873, -69.4718) (42.2722, -70.3145) (44.0967, -71.3726) (45.5838, -72.3634) (46.6185, -73.1028) (47.1314, -73.4805) knots -0.994293 -0.994293 -0.994293 -0.994293 -0.994293 -0.994293 -0.9 -0.8 -0.7 -0.6 -0.5 -0.4 -0.3 -0.2 -0.1 -0.006357 -0.006357 -0.006357 -0.006357 -0.006357 -0.006357
  line L21 (47.1314, -73.4805) -> (47.2657, -73.6356)
  line L22 (47.2657, -73.6356) -> (47.2417, -73.562)
  line L23 (47.2417, -73.562) -> (47.3061, -73.6097)
  line L24 (47.3061, -73.6097) -> (47.2073, -73.456)
  spline S6 degree 5 poles (47.2073, -73.456) (47.0161, -72.8648) (46.655, -71.6854) (46.2107, -70.0203) (45.827, -68.0395) (45.7251, -66.0044) (46.0448, -64.4455) (46.8203, -63.4254) (48.0673, -62.9624) (49.7641, -63.0312) (51.8487, -63.5828) (53.8052, -64.3705) (55.4182, -65.1396) (56.5476, -65.7243) (57.109, -66.0251) knots -0.994293 -0.994293 -0.994293 -0.994293 -0.994293 -0.994293 -0.9 -0.8 -0.7 -0.6 -0.5 -0.4 -0.3 -0.2 -0.1 -0.006357 -0.006357 -0.006357 -0.006357 -0.006357 -0.006357
  line L25 (57.109, -66.0251) -> (57.2641, -66.1595)
  line L26 (57.2641, -66.1595) -> (57.2298, -66.09)
  line L27 (57.2298, -66.09) -> (57.3003, -66.1281)
  line L28 (57.3003, -66.1281) -> (57.1807, -65.99)
  spline S7 degree 5 poles (57.1807, -65.99) (56.9073, -65.432) (56.382, -64.316) (55.7052, -62.7311) (55.0436, -60.8251) (54.6531, -58.8252) (54.7476, -57.2366) (55.3701, -56.1166) (56.5386, -55.4809) (58.2279, -55.3074) (60.3697, -55.5568) (62.4185, -56.0581) (64.1245, -56.5897) (65.3255, -57.0077) (65.9241, -57.2256) knots -0.994293 -0.994293 -0.994293 -0.994293 -0.994293 -0.994293 -0.9 -0.8 -0.7 -0.6 -0.5 -0.4 -0.3 -0.2 -0.1 -0.006357 -0.006357 -0.006357 -0.006357 -0.006357 -0.006357
  line L29 (65.9241, -57.2256) -> (66.0967, -57.3365)
  line L30 (66.0967, -57.3365) -> (66.0529, -57.2727)
  line L31 (66.0529, -57.2727) -> (66.1281, -57.3003)
  line L32 (66.1281, -57.3003) -> (65.99, -57.1807)
  spline S8 degree 5 poles (65.99, -57.1807) (65.64, -56.6673) (64.9613, -55.6374) (64.0658, -54.1649) (63.1396, -52.3725) (62.4685, -50.4485) (62.336, -48.8627) (62.7928, -47.6654) (63.8588, -46.8699) (65.5062, -46.4578) (67.6618, -46.3998) (69.761, -46.6044) (71.5254, -46.8878) (72.7737, -47.1307) (73.3971, -47.2612) knots -0.994293 -0.994293 -0.994293 -0.994293 -0.994293 -0.994293 -0.9 -0.8 -0.7 -0.6 -0.5 -0.4 -0.3 -0.2 -0.1 -0.006357 -0.006357 -0.006357 -0.006357 -0.006357 -0.006357
  line L33 (73.3971, -47.2612) -> (73.5838, -47.3464)
  line L34 (73.5838, -47.3464) -> (73.5313, -47.2894)
  line L35 (73.5313, -47.2894) -> (73.6097, -47.3061)
  line L36 (73.6097, -47.3061) -> (73.456, -47.2073)
  spline S9 degree 5 poles (73.456, -47.2073) (73.0365, -46.7489) (72.2181, -45.8261) (71.1222, -44.4961) (69.9504, -42.8537) (69.0122, -41.0448) (68.6554, -39.494) (68.9371, -38.2439) (69.8791, -37.3048) (71.4511, -36.6624) (73.5765, -36.2983) (75.6835, -36.202) (77.4702, -36.2315) (78.7403, -36.2942) (79.376, -36.3346) knots -0.994293 -0.994293 -0.994293 -0.994293 -0.994293 -0.994293 -0.9 -0.8 -0.7 -0.6 -0.5 -0.4 -0.3 -0.2 -0.1 -0.006357 -0.006357 -0.006357 -0.006357 -0.006357 -0.006357
  line L37 (79.376, -36.3346) -> (79.5729, -36.3924)
  line L38 (79.5729, -36.3924) -> (79.5128, -36.3435)
  line L39 (79.5128, -36.3435) -> (79.5928, -36.3488)
  line L40 (79.5928, -36.3488) -> (79.4266, -36.2729)
  spline S10 degree 5 poles (79.4266, -36.2729) (78.9461, -35.8789) (78.0047, -35.082) (76.7307, -33.9214) (75.3371, -32.4625) (74.151, -30.8056) (73.5772, -29.3213) (73.6781, -28.0438) (74.4769, -26.9802) (75.9415, -26.1207) (77.9934, -25.4578) (80.0652, -25.0626) (81.8379, -24.8375) (83.1041, -24.7188) (83.7391, -24.6684) knots -0.994293 -0.994293 -0.994293 -0.994293 -0.994293 -0.994293 -0.9 -0.8 -0.7 -0.6 -0.5 -0.4 -0.3 -0.2 -0.1 -0.006357 -0.006357 -0.006357 -0.006357 -0.006357 -0.006357
  line L41 (83.7391, -24.6684) -> (83.9421, -24.6976)
  line L42 (83.9421, -24.6976) -> (83.8757, -24.6577)
  line L43 (83.8757, -24.6577) -> (83.9556, -24.6516)
  line L44 (83.9556, -24.6516) -> (83.7803, -24.6001)
  spline S11 degree 5 poles (83.7803, -24.6001) (83.2487, -24.2785) (82.2035, -23.6237) (80.7772, -22.6562) (79.1902, -21.4105) (77.7804, -19.9392) (77.0011, -18.5517) (76.9192, -17.2729) (77.5585, -16.1064) (78.8858, -15.0472) (80.8225, -14.099) (82.817, -13.4131) (84.5397, -12.938) (85.776, -12.6403) (86.3974, -12.5) knots -0.994293 -0.994293 -0.994293 -0.994293 -0.994293 -0.994293 -0.9 -0.8 -0.7 -0.6 -0.5 -0.4 -0.3 -0.2 -0.1 -0.006357 -0.006357 -0.006357 -0.006357 -0.006357 -0.006357
  line L45 (86.3974, -12.5) -> (86.6025, -12.5)
  line L46 (86.6025, -12.5) -> (86.5312, -12.47)
  line L47 (86.5312, -12.47) -> (86.6094, -12.4525)
  line L48 (86.6094, -12.4525) -> (86.4285, -12.4265)
  spline S12 degree 5 poles (86.4285, -12.4265) (85.8565, -12.1839) (84.7287, -11.6844) (83.1793, -10.9298) (81.4312, -9.9227) (79.8263, -8.667) (78.8575, -7.4045) (78.5945, -6.1503) (79.0612, -4.9048) (80.2243, -3.6674) (82.0064, -2.4533) (83.883, -1.4905) (85.5204, -0.775) (86.7019, -0.3044) (87.2969, -0.0771) knots -0.994293 -0.994293 -0.994293 -0.994293 -0.994293 -0.994293 -0.9 -0.8 -0.7 -0.6 -0.5 -0.4 -0.3 -0.2 -0.1 -0.006357 -0.006357 -0.006357 -0.006357 -0.006357 -0.006357
  line L49 (87.2969, -0.0771) -> (87.5, -0.0479)
  line L50 (87.5, -0.0479) -> (87.4251, -0.0284)
  line L51 (87.4251, -0.0284) -> (87.5, 0)
  line L52 (87.5, 0) -> (87.3173, 0)
  spline S13 degree 5 poles (87.3173, 0) (86.7166, 0.1588) (85.5292, 0.4926) (83.8882, 1.0191) (82.0144, 1.7672) (80.2473, 2.7817) (79.1086, 3.8935) (78.6698, 5.0974) (78.9545, 6.3967) (79.9297, 7.787) (81.5208, 9.2424) (83.2413, 10.4625) (84.7603, 11.4037) (85.8627, 12.0376) (86.4193, 12.3473) knots -0.994293 -0.994293 -0.994293 -0.994293 -0.994293 -0.994293 -0.9 -0.8 -0.7 -0.6 -0.5 -0.4 -0.3 -0.2 -0.1 -0.006357 -0.006357 -0.006357 -0.006357 -0.006357 -0.006357
  line L53 (86.4193, 12.3473) -> (86.6162, 12.4051)
  line L54 (86.6162, 12.4051) -> (86.5392, 12.4138)
  line L55 (86.5392, 12.4138) -> (86.6094, 12.4525)
  line L56 (86.6094, 12.4525) -> (86.4285, 12.4265)
  spline S14 degree 5 poles (86.4285, 12.4265) (85.8113, 12.4982) (84.5885, 12.6597) (82.8893, 12.9472) (80.9282, 13.4211) (79.0346, 14.1738) (77.7493, 15.1122) (77.1436, 16.2414) (77.2405, 17.568) (78.0079, 19.0829) (79.3757, 20.75) (80.905, 22.2025) (82.2746, 23.3503) (83.2756, 24.1346) (83.7825, 24.5204) knots -0.994293 -0.994293 -0.994293 -0.994293 -0.994293 -0.994293 -0.9 -0.8 -0.7 -0.6 -0.5 -0.4 -0.3 -0.2 -0.1 -0.006357 -0.006357 -0.006357 -0.006357 -0.006357 -0.006357
  line L57 (83.7825, 24.5204) -> (83.9691, 24.6056)
  line L58 (83.9691, 24.6056) -> (83.8917, 24.6033)
  line L59 (83.8917, 24.6033) -> (83.9556, 24.6516)
  line L60 (83.9556, 24.6516) -> (83.7803, 24.6001)
  spline S15 degree 5 poles (83.7803, 24.6001) (83.1592, 24.5832) (81.9259, 24.569) (80.203, 24.6118) (78.1944, 24.8018) (76.213, 25.2773) (74.8073, 26.0232) (74.047, 27.0548) (73.9542, 28.3817) (74.4981, 29.9904) (75.6147, 31.8351) (76.9218, 33.4905) (78.1141, 34.8215) (78.9933, 35.7403) (79.4401, 36.1943) knots -0.994293 -0.994293 -0.994293 -0.994293 -0.994293 -0.994293 -0.9 -0.8 -0.7 -0.6 -0.5 -0.4 -0.3 -0.2 -0.1 -0.006357 -0.006357 -0.006357 -0.006357 -0.006357 -0.006357
  line L61 (79.4401, 36.1943) -> (79.6127, 36.3052)
  line L62 (79.6127, 36.3052) -> (79.5364, 36.2919)
  line L63 (79.5364, 36.2919) -> (79.5928, 36.3488)
  line L64 (79.5928, 36.3488) -> (79.4266, 36.2729)
  spline S16 degree 5 poles (79.4266, 36.2729) (78.8142, 36.1678) (77.5954, 35.9782) (75.884, 35.7754) (73.8688, 35.6775) (71.8399, 35.8663) (70.3423, 36.4045) (69.443, 37.3174) (69.1623, 38.6176) (69.4718, 40.2873) (70.3145, 42.2722) (71.3726, 44.0967) (72.3634, 45.5838) (73.1028, 46.6185) (73.4805, 47.1314) knots -0.994293 -0.994293 -0.994293 -0.994293 -0.994293 -0.994293 -0.9 -0.8 -0.7 -0.6 -0.5 -0.4 -0.3 -0.2 -0.1 -0.006357 -0.006357 -0.006357 -0.006357 -0.006357 -0.006357
  line L65 (73.4805, 47.1314) -> (73.6356, 47.2657)
  line L66 (73.6356, 47.2657) -> (73.562, 47.2417)
  line L67 (73.562, 47.2417) -> (73.6097, 47.3061)
  line L68 (73.6097, 47.3061) -> (73.456, 47.2073)
  spline S17 degree 5 poles (73.456, 47.2073) (72.8648, 47.0161) (71.6854, 46.655) (70.0203, 46.2107) (68.0395, 45.827) (66.0044, 45.7251) (64.4455, 46.0448) (63.4254, 46.8203) (62.9624, 48.0673) (63.0312, 49.7641) (63.5828, 51.8487) (64.3705, 53.8052) (65.1396, 55.4182) (65.7243, 56.5476) (66.0251, 57.109) knots -0.994293 -0.994293 -0.994293 -0.994293 -0.994293 -0.994293 -0.9 -0.8 -0.7 -0.6 -0.5 -0.4 -0.3 -0.2 -0.1 -0.006357 -0.006357 -0.006357 -0.006357 -0.006357 -0.006357
  line L69 (66.0251, 57.109) -> (66.1595, 57.2641)
  line L70 (66.1595, 57.2641) -> (66.09, 57.2298)
  line L71 (66.09, 57.2298) -> (66.1281, 57.3003)
  line L72 (66.1281, 57.3003) -> (65.99, 57.1807)
  spline S18 degree 5 poles (65.99, 57.1807) (65.432, 56.9073) (64.316, 56.382) (62.7311, 55.7052) (60.8251, 55.0436) (58.8252, 54.6531) (57.2366, 54.7476) (56.1166, 55.3701) (55.4809, 56.5386) (55.3074, 58.2279) (55.5568, 60.3697) (56.0581, 62.4185) (56.5897, 64.1245) (57.0077, 65.3255) (57.2256, 65.9241) knots -0.994293 -0.994293 -0.994293 -0.994293 -0.994293 -0.994293 -0.9 -0.8 -0.7 -0.6 -0.5 -0.4 -0.3 -0.2 -0.1 -0.006357 -0.006357 -0.006357 -0.006357 -0.006357 -0.006357
  line L73 (57.2256, 65.9241) -> (57.3365, 66.0967)
  line L74 (57.3365, 66.0967) -> (57.2727, 66.0529)
  line L75 (57.2727, 66.0529) -> (57.3003, 66.1281)
  line L76 (57.3003, 66.1281) -> (57.1807, 65.99)
  spline S19 degree 5 poles (57.1807, 65.99) (56.6673, 65.64) (55.6374, 64.9613) (54.1649, 64.0658) (52.3725, 63.1396) (50.4485, 62.4685) (48.8627, 62.336) (47.6654, 62.7928) (46.8699, 63.8588) (46.4578, 65.5062) (46.3998, 67.6618) (46.6044, 69.761) (46.8878, 71.5254) (47.1307, 72.7737) (47.2612, 73.3971) knots -0.994293 -0.994293 -0.994293 -0.994293 -0.994293 -0.994293 -0.9 -0.8 -0.7 -0.6 -0.5 -0.4 -0.3 -0.2 -0.1 -0.006357 -0.006357 -0.006357 -0.006357 -0.006357 -0.006357
  line L77 (47.2612, 73.3971) -> (47.3464, 73.5838)
  line L78 (47.3464, 73.5838) -> (47.2894, 73.5313)
  line L79 (47.2894, 73.5313) -> (47.3061, 73.6097)
  line L80 (47.3061, 73.6097) -> (47.2073, 73.456)
  spline S20 degree 5 poles (47.2073, 73.456) (46.7489, 73.0365) (45.8261, 72.2181) (44.4961, 71.1222) (42.8537, 69.9504) (41.0448, 69.0122) (39.494, 68.6554) (38.2439, 68.9371) (37.3048, 69.8791) (36.6624, 71.4511) (36.2983, 73.5765) (36.202, 75.6835) (36.2315, 77.4702) (36.2942, 78.7403) (36.3346, 79.376) knots -0.994293 -0.994293 -0.994293 -0.994293 -0.994293 -0.994293 -0.9 -0.8 -0.7 -0.6 -0.5 -0.4 -0.3 -0.2 -0.1 -0.006357 -0.006357 -0.006357 -0.006357 -0.006357 -0.006357
  line L81 (36.3346, 79.376) -> (36.3924, 79.5729)
  line L82 (36.3924, 79.5729) -> (36.3435, 79.5128)
  line L83 (36.3435, 79.5128) -> (36.3488, 79.5928)
  line L84 (36.3488, 79.5928) -> (36.2729, 79.4266)
  spline S21 degree 5 poles (36.2729, 79.4266) (35.8789, 78.9461) (35.082, 78.0047) (33.9214, 76.7307) (32.4625, 75.3371) (30.8056, 74.151) (29.3213, 73.5772) (28.0438, 73.6781) (26.9802, 74.4769) (26.1207, 75.9415) (25.4578, 77.9934) (25.0626, 80.0652) (24.8375, 81.8379) (24.7188, 83.1041) (24.6684, 83.7391) knots -0.994293 -0.994293 -0.994293 -0.994293 -0.994293 -0.994293 -0.9 -0.8 -0.7 -0.6 -0.5 -0.4 -0.3 -0.2 -0.1 -0.006357 -0.006357 -0.006357 -0.006357 -0.006357 -0.006357
  line L85 (24.6684, 83.7391) -> (24.6976, 83.9421)
  line L86 (24.6976, 83.9421) -> (24.6577, 83.8757)
  line L87 (24.6577, 83.8757) -> (24.6516, 83.9556)
  line L88 (24.6516, 83.9556) -> (24.6001, 83.7803)
  spline S22 degree 5 poles (24.6001, 83.7803) (24.2785, 83.2487) (23.6237, 82.2035) (22.6562, 80.7772) (21.4105, 79.1902) (19.9392, 77.7804) (18.5517, 77.0011) (17.2729, 76.9192) (16.1064, 77.5585) (15.0472, 78.8858) (14.099, 80.8225) (13.4131, 82.817) (12.938, 84.5397) (12.6403, 85.776) (12.5, 86.3974) knots -0.994293 -0.994293 -0.994293 -0.994293 -0.994293 -0.994293 -0.9 -0.8 -0.7 -0.6 -0.5 -0.4 -0.3 -0.2 -0.1 -0.006357 -0.006357 -0.006357 -0.006357 -0.006357 -0.006357
  line L89 (12.5, 86.3974) -> (12.5, 86.6025)
  line L90 (12.5, 86.6025) -> (12.47, 86.5312)
  line L91 (12.47, 86.5312) -> (12.4525, 86.6094)
  line L92 (12.4525, 86.6094) -> (12.4265, 86.4285)
  spline S23 degree 5 poles (12.4265, 86.4285) (12.1839, 85.8565) (11.6844, 84.7287) (10.9298, 83.1793) (9.9227, 81.4312) (8.667, 79.8263) (7.4045, 78.8575) (6.1503, 78.5945) (4.9048, 79.0612) (3.6674, 80.2243) (2.4533, 82.0064) (1.4905, 83.883) (0.775, 85.5204) (0.3044, 86.7019) (0.0771, 87.2969) knots -0.994293 -0.994293 -0.994293 -0.994293 -0.994293 -0.994293 -0.9 -0.8 -0.7 -0.6 -0.5 -0.4 -0.3 -0.2 -0.1 -0.006357 -0.006357 -0.006357 -0.006357 -0.006357 -0.006357
  line L93 (0.0771, 87.2969) -> (0.0479, 87.5)
  line L94 (0.0479, 87.5) -> (0.0284, 87.4251)
  line L95 (0.0284, 87.4251) -> (0, 87.5)
  line L96 (0, 87.5) -> (0, 87.3173)
  spline S24 degree 5 poles (0, 87.3173) (-0.1588, 86.7166) (-0.4926, 85.5292) (-1.0191, 83.8882) (-1.7672, 82.0144) (-2.7817, 80.2473) (-3.8935, 79.1086) (-5.0974, 78.6698) (-6.3967, 78.9545) (-7.787, 79.9297) (-9.2424, 81.5208) (-10.4625, 83.2413) (-11.4037, 84.7603) (-12.0376, 85.8627) (-12.3473, 86.4193) knots -0.994293 -0.994293 -0.994293 -0.994293 -0.994293 -0.994293 -0.9 -0.8 -0.7 -0.6 -0.5 -0.4 -0.3 -0.2 -0.1 -0.006357 -0.006357 -0.006357 -0.006357 -0.006357 -0.006357
  line L97 (-12.3473, 86.4193) -> (-12.4051, 86.6162)
  line L98 (-12.4051, 86.6162) -> (-12.4138, 86.5392)
  line L99 (-12.4138, 86.5392) -> (-12.4525, 86.6094)
  line L100 (-12.4525, 86.6094) -> (-12.4265, 86.4285)
  spline S25 degree 5 poles (-12.4265, 86.4285) (-12.4982, 85.8113) (-12.6597, 84.5885) (-12.9472, 82.8893) (-13.4211, 80.9282) (-14.1738, 79.0346) (-15.1122, 77.7493) (-16.2414, 77.1436) (-17.568, 77.2405) (-19.0829, 78.0079) (-20.75, 79.3757) (-22.2025, 80.905) (-23.3503, 82.2746) (-24.1346, 83.2756) (-24.5204, 83.7825) knots -0.994293 -0.994293 -0.994293 -0.994293 -0.994293 -0.994293 -0.9 -0.8 -0.7 -0.6 -0.5 -0.4 -0.3 -0.2 -0.1 -0.006357 -0.006357 -0.006357 -0.006357 -0.006357 -0.006357
  line L101 (-24.5204, 83.7825) -> (-24.6056, 83.9691)
  line L102 (-24.6056, 83.9691) -> (-24.6033, 83.8917)
  line L103 (-24.6033, 83.8917) -> (-24.6516, 83.9556)
  line L104 (-24.6516, 83.9556) -> (-24.6001, 83.7803)
  spline S26 degree 5 poles (-24.6001, 83.7803) (-24.5832, 83.1592) (-24.569, 81.9259) (-24.6118, 80.203) (-24.8018, 78.1944) (-25.2773, 76.213) (-26.0232, 74.8073) (-27.0548, 74.047) (-28.3817, 73.9542) (-29.9904, 74.4981) (-31.8351, 75.6147) (-33.4905, 76.9218) (-34.8215, 78.1141) (-35.7403, 78.9933) (-36.1943, 79.4401) knots -0.994293 -0.994293 -0.994293 -0.994293 -0.994293 -0.994293 -0.9 -0.8 -0.7 -0.6 -0.5 -0.4 -0.3 -0.2 -0.1 -0.006357 -0.006357 -0.006357 -0.006357 -0.006357 -0.006357
  line L105 (-36.1943, 79.4401) -> (-36.3052, 79.6127)
  line L106 (-36.3052, 79.6127) -> (-36.2919, 79.5364)
  line L107 (-36.2919, 79.5364) -> (-36.3488, 79.5928)
  line L108 (-36.3488, 79.5928) -> (-36.2729, 79.4266)
  spline S27 degree 5 poles (-36.2729, 79.4266) (-36.1678, 78.8142) (-35.9782, 77.5954) (-35.7754, 75.884) (-35.6775, 73.8688) (-35.8663, 71.8399) (-36.4045, 70.3423) (-37.3174, 69.443) (-38.6176, 69.1623) (-40.2873, 69.4718) (-42.2722, 70.3145) (-44.0967, 71.3726) (-45.5838, 72.3634) (-46.6185, 73.1028) (-47.1314, 73.4805) knots -0.994293 -0.994293 -0.994293 -0.994293 -0.994293 -0.994293 -0.9 -0.8 -0.7 -0.6 -0.5 -0.4 -0.3 -0.2 -0.1 -0.006357 -0.006357 -0.006357 -0.006357 -0.006357 -0.006357
  line L109 (-47.1314, 73.4805) -> (-47.2657, 73.6356)
  line L110 (-47.2657, 73.6356) -> (-47.2417, 73.562)
  line L111 (-47.2417, 73.562) -> (-47.3061, 73.6097)
  line L112 (-47.3061, 73.6097) -> (-47.2073, 73.456)
  spline S28 degree 5 poles (-47.2073, 73.456) (-47.0161, 72.8648) (-46.655, 71.6854) (-46.2107, 70.0203) (-45.827, 68.0395) (-45.7251, 66.0044) (-46.0448, 64.4455) (-46.8203, 63.4254) (-48.0673, 62.9624) (-49.7641, 63.0312) (-51.8487, 63.5828) (-53.8052, 64.3705) (-55.4182, 65.1396) (-56.5476, 65.7243) (-57.109, 66.0251) knots -0.994293 -0.994293 -0.994293 -0.994293 -0.994293 -0.994293 -0.9 -0.8 -0.7 -0.6 -0.5 -0.4 -0.3 -0.2 -0.1 -0.006357 -0.006357 -0.006357 -0.006357 -0.006357 -0.006357
  line L113 (-57.109, 66.0251) -> (-57.2641, 66.1595)
  line L114 (-57.2641, 66.1595) -> (-57.2298, 66.09)
  line L115 (-57.2298, 66.09) -> (-57.3003, 66.1281)
  line L116 (-57.3003, 66.1281) -> (-57.1807, 65.99)
  spline S29 degree 5 poles (-57.1807, 65.99) (-56.9073, 65.432) (-56.382, 64.316) (-55.7052, 62.7311) (-55.0436, 60.8251) (-54.6531, 58.8252) (-54.7476, 57.2366) (-55.3701, 56.1166) (-56.5386, 55.4809) (-58.2279, 55.3074) (-60.3697, 55.5568) (-62.4185, 56.0581) (-64.1245, 56.5897) (-65.3255, 57.0077) (-65.9241, 57.2256) knots -0.994293 -0.994293 -0.994293 -0.994293 -0.994293 -0.994293 -0.9 -0.8 -0.7 -0.6 -0.5 -0.4 -0.3 -0.2 -0.1 -0.006357 -0.006357 -0.006357 -0.006357 -0.006357 -0.006357
  line L117 (-65.9241, 57.2256) -> (-66.0967, 57.3365)
  line L118 (-66.0967, 57.3365) -> (-66.0529, 57.2727)
  line L119 (-66.0529, 57.2727) -> (-66.1281, 57.3003)
  line L120 (-66.1281, 57.3003) -> (-65.99, 57.1807)
  spline S30 degree 5 poles (-65.99, 57.1807) (-65.64, 56.6673) (-64.9613, 55.6374) (-64.0658, 54.1649) (-63.1396, 52.3725) (-62.4685, 50.4485) (-62.336, 48.8627) (-62.7928, 47.6654) (-63.8588, 46.8699) (-65.5062, 46.4578) (-67.6618, 46.3998) (-69.761, 46.6044) (-71.5254, 46.8878) (-72.7737, 47.1307) (-73.3971, 47.2612) knots -0.994293 -0.994293 -0.994293 -0.994293 -0.994293 -0.994293 -0.9 -0.8 -0.7 -0.6 -0.5 -0.4 -0.3 -0.2 -0.1 -0.006357 -0.006357 -0.006357 -0.006357 -0.006357 -0.006357
  line L121 (-73.3971, 47.2612) -> (-73.5838, 47.3464)
  line L122 (-73.5838, 47.3464) -> (-73.5313, 47.2894)
  line L123 (-73.5313, 47.2894) -> (-73.6097, 47.3061)
  line L124 (-73.6097, 47.3061) -> (-73.456, 47.2073)
  spline S31 degree 5 poles (-73.456, 47.2073) (-73.0365, 46.7489) (-72.2181, 45.8261) (-71.1222, 44.4961) (-69.9504, 42.8537) (-69.0122, 41.0448) (-68.6554, 39.494) (-68.9371, 38.2439) (-69.8791, 37.3048) (-71.4511, 36.6624) (-73.5765, 36.2983) (-75.6835, 36.202) (-77.4702, 36.2315) (-78.7403, 36.2942) (-79.376, 36.3346) knots -0.994293 -0.994293 -0.994293 -0.994293 -0.994293 -0.994293 -0.9 -0.8 -0.7 -0.6 -0.5 -0.4 -0.3 -0.2 -0.1 -0.006357 -0.006357 -0.006357 -0.006357 -0.006357 -0.006357
  line L125 (-79.376, 36.3346) -> (-79.5729, 36.3924)
  line L126 (-79.5729, 36.3924) -> (-79.5128, 36.3435)
  line L127 (-79.5128, 36.3435) -> (-79.5928, 36.3488)
  line L128 (-79.5928, 36.3488) -> (-79.4266, 36.2729)
  spline S32 degree 5 poles (-79.4266, 36.2729) (-78.9461, 35.8789) (-78.0047, 35.082) (-76.7307, 33.9214) (-75.3371, 32.4625) (-74.151, 30.8056) (-73.5772, 29.3213) (-73.6781, 28.0438) (-74.4769, 26.9802) (-75.9415, 26.1207) (-77.9934, 25.4578) (-80.0652, 25.0626) (-81.8379, 24.8375) (-83.1041, 24.7188) (-83.7391, 24.6684) knots -0.994293 -0.994293 -0.994293 -0.994293 -0.994293 -0.994293 -0.9 -0.8 -0.7 -0.6 -0.5 -0.4 -0.3 -0.2 -0.1 -0.006357 -0.006357 -0.006357 -0.006357 -0.006357 -0.006357
  line L129 (-83.7391, 24.6684) -> (-83.9421, 24.6976)
  line L130 (-83.9421, 24.6976) -> (-83.8757, 24.6577)
  line L131 (-83.8757, 24.6577) -> (-83.9556, 24.6516)
  line L132 (-83.9556, 24.6516) -> (-83.7803, 24.6001)